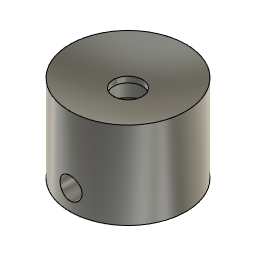
EggBot Egg Mount 20-15-5 (Autodesk Fusion 360 design; units mm, degrees)
Autodesk Fusion 360 part; units mm, degrees
sketch "Sketch1" plane through (0, 0, 0) normal (1, 0, 0) x (0, 1, 0)
  line L0 (0, 0) -> (10, 0)
  line L1 (10, 0) -> (10, 15)
  line L2 (2.5, 13.4762) -> (2.5, 12.4762)
  line L3 (2.5, 12.4762) -> (5, 12.4762)
  line L4 (5, 12.4762) -> (5, 8.4762)
  line L5 (5, 8.4762) -> (2.75, 8.4762)
  line L6 (2.75, 8.4762) -> (2.75, 0)
  line L7 (0, 0) -> (0, 15) construction
  line L8 (0, 15) -> (0, 45) construction
  arc A0 (2.5, 13.4762) -> (10, 15) centre (0, 45) ccw
  dimension "d1" = 10
  dimension "d3" = 2.75
  dimension "d4" = 2.5
  dimension "d5" = 4
  dimension "d6" = 1
  dimension "d8" = 30
  dimension "d9" = 15
  dimension "d10" = 5
  constraint coincident L0.start L7.start
  constraint horizontal L0
  constraint perpendicular L0 L1
  constraint parallel L1 L2
  constraint perpendicular L2 L3
  constraint perpendicular L3 L4
  constraint perpendicular L4 L5
  constraint coincident L0 L6.end
  constraint perpendicular L0 L6
  constraint perpendicular L0 L7
  constraint perpendicular L0 L8
  constraint equal L1 L7
  constraint coincident L2 A0.start
  constraint coincident L8.end A0.centre
  constraint coincident L2.start A0.start
  measures "d1" distance of L0.start L0.end
  measures "d3" distance of L0.start L6.end
  measures "d4" horizontal distance of L0.start L2.end
  measures "d5" distance of L3.end L4.end
  measures "d6" distance of L2.start L2.end
  measures "d8" distance of L7.end L8.end
  measures "d9" distance of L0.start L7.end
  measures "d10" distance of L3.end L7
revolve "Revolve1" add sketch "Sketch1" angle 360 about axis through (0, 0, 0) along (0, 0, 1)
sketch "Sketch2" plane through (0, 0, 0) normal (0, 1, 0) x (1, 0, 0)
  circle A0 centre (0, -3.5) radius 1.9
  dimension "d12" = 3.8
  dimension "d13" = 3.5
  measures "d12" diameter of A0
  measures "d13" distance of origin A0.centre
extrude "Extrude1" cut sketch "Sketch2" against normal through all
sketch "Sketch3" plane through (0, 0, 0) normal (0, 0, -1) x (1, 0, 0)
  circle A0 centre (0, 0) radius 10
  circle A1 centre (0, 0) radius 2.75
  line L0 (2.9994, 3.75) -> (-3.0006, 3.75)
  line L1 (-3.0006, 3.75) -> (-3.0006, 6.75)
  line L2 (-3.0006, 6.75) -> (2.9994, 6.75)
  line L3 (2.9994, 6.75) -> (2.9994, 3.75)
  line L4 (2.9994, 3.75) -> (-3.0006, 6.75) construction
  line L5 (-3.0006, 3.75) -> (2.9994, 6.75) construction
  line L6 (-0.0006, 3.75) -> (-0.0006, 2.75) construction
  point P0 (-0.0006, 5.25)
  point P1 (-0.0006, 5.25)
  dimension "d15" = 6
  dimension "d16" = 3
  dimension "d22" = 1
  constraint perpendicular L0 L1
  constraint parallel L0 L2
  constraint parallel L1 L3
  constraint horizontal L0
  constraint coincident L4 P1
  constraint coincident L5 P1
  constraint coincident P1 P0
  constraint midpoint L0 L6.start
  constraint coincident A1 L6.end
  constraint perpendicular L0 L6
  measures "d15" distance of L1.end L2.end
  measures "d16" distance of L0.end L1.end
  measures "d22" distance of L6.start L6.end
extrude "Extrude2" cut sketch "Sketch3" against normal blind 7.5 contours L0 L1 L2 L3
equation "d1 = Diameter / 2"
equation "d3 = ( RodDiameter + 0.5 mm ) / 2"
equation "d9 = Length"
equation "d17 = -( d13 * 2 + 0.5 mm )"
equation "Diameter = 20 mm"
equation "Length = 15 mm"
equation "RodDiameter = 5 mm"
